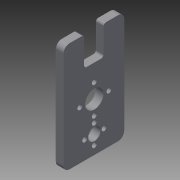
# Autodesk Inventor part: carriage
Saved by Autodesk Inventor 2015 SP1 (Build 190203100, 203)
## iProperties
Created: 2016-07-08
Part Number: carriage
Material: Generic
Document SubType Name: Modeling
Designer: lustinga
Density: 1 g/cm^3
Appearance: Default
Mass: 16.9887 g
Surface Area: 124.024 cm^2
Volume: 16.9887 cm^3
Author: lustinga
Autodesk Inventor part; units mm, degrees
ref_plane "YZ Plane" through (0, 0, 0) normal (1, 0, 0) x (0, 1, 0)
ref_plane "XZ Plane" through (0, 0, 0) normal (0, 1, 0) x (-1, 0, 0)
ref_plane "XY Plane" through (0, 0, 0) normal (0, 0, 1) x (1, 0, 0)
sketch "Sketch1" plane through (0, 0, 0) normal (1, 0, 0) x (0, 1, 0)
  line L0 (-116.4234, 72.9982) -> (-116.4234, -7.0018)
  line L1 (-111.4234, -12.0018) -> (-86.4234, -12.0018)
  line L2 (-81.4234, -7.0018) -> (-81.4234, 72.9982)
  line L3 (-90.9234, 75.9982) -> (-90.9234, 55.9982)
  line L4 (-92.9234, 53.9982) -> (-104.9234, 53.9982)
  line L5 (-106.9234, 55.9982) -> (-106.9234, 75.9982)
  line L6 (-86.4234, 77.9982) -> (-88.9234, 77.9982)
  line L7 (-108.9234, 77.9982) -> (-111.4234, 77.9982)
  circle A0 centre (-98.1419, 27.9982) radius 7.5
  circle A1 centre (-98.1419, 2.9982) radius 5.1
  circle A2 centre (-110.1419, 27.9982) radius 2
  circle A3 centre (-112.4234, 61.8916) radius 2
  circle A4 centre (-56.4234, 61.8916) radius 2
  circle A5 centre (-106.1419, 2.9982) radius 2
  circle A6 centre (-98.1419, 15.9982) radius 2
  circle A7 centre (-86.1419, 27.9982) radius 2
  circle A8 centre (-98.1419, 39.9982) radius 2
  circle A9 centre (-98.1419, -5.0018) radius 2
  circle A10 centre (-90.1419, 2.9982) radius 2
  circle A11 centre (-98.1419, 10.9982) radius 2
  arc A12 (-111.4234, 77.9982) -> (-116.4234, 72.9982) centre (-111.4234, 72.9982) ccw
  arc A13 (-81.4234, 72.9982) -> (-86.4234, 77.9982) centre (-86.4234, 72.9982) ccw
  arc A14 (-116.4234, -7.0018) -> (-111.4234, -12.0018) centre (-111.4234, -7.0018) ccw
  arc A15 (-86.4234, -12.0018) -> (-81.4234, -7.0018) centre (-86.4234, -7.0018) ccw
  arc A16 (-106.9234, 55.9982) -> (-104.9234, 53.9982) centre (-104.9234, 55.9982) ccw
  arc A17 (-92.9234, 53.9982) -> (-90.9234, 55.9982) centre (-92.9234, 55.9982) ccw
  arc A18 (-106.9234, 75.9982) -> (-108.9234, 77.9982) centre (-108.9234, 75.9982) ccw
  arc A19 (-88.9234, 77.9982) -> (-90.9234, 75.9982) centre (-88.9234, 75.9982) ccw
  point P0 (-81.4234, 77.9982)
  point P1 (-116.4234, -12.0018)
  point P2 (-116.4234, 77.9982)
  point P3 (-81.4234, -12.0018)
  point P4 (-90.9234, 77.9982)
  point P5 (-90.9234, 53.9982)
  point P6 (-106.9234, 53.9982)
  point P7 (-106.9234, 77.9982)
  dimension "d29" = 360
  dimension "d44" = 35
  dimension "d45" = 90
  dimension "d46" = 16
  dimension "d47" = 24
  dimension "d48" = 15
  dimension "d53" = 10.2
  dimension "d54" = 25
  dimension "d55" = 26
  dimension "d58" = 56
  dimension "d59" = 4
  dimension "d60" = 4
  dimension "d62" = 12
  dimension "d63" = 8
  dimension "d66" = 360
  dimension "d70" = 360
  dimension "d72" = 5
  dimension "d73" = 2
  constraints: 20 centre point, 16 end point, 16 point on circle, 16 point on line, 16 tangent, 9 equal radius, 5 perpendicular, 3 parallel, 2 equal length, 2 horizontal, 1 horizontal alignment, 1 vertical, 18 other
  measures "d44" distance of point (-81.423, -12.002) point (-116.423, -12.002)
  measures "d45" distance of point (-116.423, -12.002) point (-116.423, 77.998)
  measures "d46" distance of point (-90.923, 53.998) point (-106.923, 53.998)
  measures "d47" distance of point (-90.923, 77.998) point (-90.923, 53.998)
  measures "d48" diameter of A0
  measures "d53" diameter of A1
  measures "d54" distance of A0.centre A1.centre
  measures "d55" distance from line of L4 A0.centre
  measures "d58" distance of A4.centre A3.centre
  measures "d59" distance from line of L0 A3.centre
  measures "d60" diameter of A3
  measures "d62" distance of A0.centre A2.centre
  measures "d63" distance of A1.centre A5.centre
  measures "d72" radius of A12
  measures "d73" radius of A16
extrude "Extrusion1" add sketch "Sketch1" along normal blind 6.35 contours A12 L7 A18 L5 A16 L4 A17 L3 A19 L6 A13 L2 A15 L1 A14 L0 | A3 | A6 | A11
body "Solid1"
